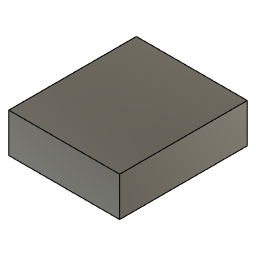
ConsoleFrame v17 (Autodesk Fusion 360 archive; units mm, degrees)
design "DAC Mock"
Autodesk Fusion 360 part; units mm, degrees
sketch "Sketch1" plane through (0, 0, 0) normal (0, 0, 1) x (1, 0, 0)
  line L0 (0, 0) -> (0, 65)
  line L1 (0, 65) -> (56.5, 65)
  line L2 (56.5, 65) -> (56.5, 0)
  line L3 (56.5, 0) -> (0, 0)
  dimension "d1" = 65
  dimension "d2" = 56.5
  constraint coincident L0.start L3.end
  constraint vertical L0
  constraint perpendicular L0 L1
  constraint perpendicular L1 L2
  constraint perpendicular L0 L3
  measures "d1" distance of L0.start L0.end
  measures "d2" distance of L0.end L1.end
extrude "Extrude1" add sketch "Sketch1" along normal blind 20

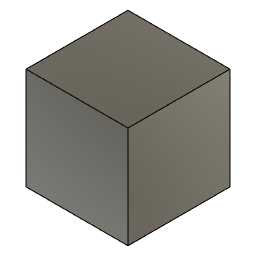
design "Relay Block"
Autodesk Fusion 360 part; units mm, degrees
sketch "Sketch1" plane through (0, 0, 0) normal (0, 0, 1) x (1, 0, 0)
  line L0 (0, 0) -> (0, 30)
  line L1 (0, 30) -> (30, 30)
  line L2 (30, 30) -> (30, 0)
  line L3 (30, 0) -> (0, 0)
  dimension "d1" = 30
  dimension "d2" = 30
  constraint coincident L0.start L3.end
  constraint vertical L0
  constraint perpendicular L0 L1
  constraint perpendicular L1 L2
  constraint perpendicular L0 L3
  measures "d1" distance of L0.start L0.end
  measures "d2" distance of L0.end L1.end
extrude "Extrude1" add sketch "Sketch1" along normal blind 30

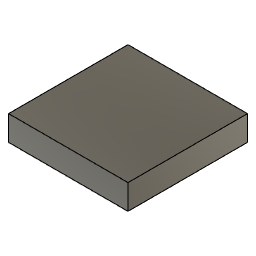
design "FanBlock"
Autodesk Fusion 360 part; units mm, degrees
sketch "Sketch1" plane through (0, 0, 0) normal (0, 0, 1) x (1, 0, 0)
  line L0 (0, 0) -> (0, 60) construction
  line L1 (0, 0) -> (60, 0) construction
  line L2 (0, 0) -> (-60, 0) construction
  line L3 (0, 60) -> (-60, 60)
  line L4 (-60, 60) -> (-60, -60)
  line L5 (-60, -60) -> (60, -60)
  line L6 (-60, 60) -> (60, 60)
  line L7 (60, 60) -> (60, -60)
  dimension "d1" = 60
  dimension "d2" = 60
  dimension "d3" = 60
  dimension "d4" = 120
  dimension "d5" = 120
  dimension "d6" = 120
  constraint coincident L0.start L1.start
  constraint vertical L0
  constraint perpendicular L0 L1
  constraint perpendicular L0 L2
  constraint perpendicular L0 L3
  constraint perpendicular L2 L4
  constraint horizontal L5
  constraint perpendicular L4 L6
  measures "d1" distance of L0.start L0.end
  measures "d2" distance of L0.start L1.end
  measures "d3" distance of L0.start L2.end
  measures "d4" distance of L3.end L4.end
  measures "d5" distance of L4.end L5.end
  measures "d6" distance of L3.end L6.end
extrude "Extrude1" add sketch "Sketch1" along normal blind 25

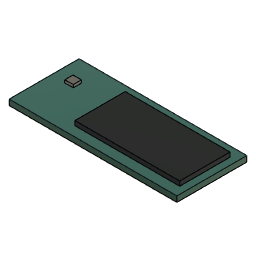
design "Adatrinket Power control"
Autodesk Fusion 360 part; units mm, degrees
sketch "Sketch1" plane through (0, 0, 0) normal (0, 0, 1) x (1, 0, 0)
  line L0 (0, 0) -> (0, 18)
  line L1 (0, 0) -> (37.5, 0)
  line L2 (0, 18) -> (37.5, 18)
  line L3 (37.5, 18) -> (37.5, 0)
  dimension "d1" = 18
  dimension "d2" = 37.5
  dimension "d3" = 37.5
  constraint coincident L0.start L1.start
  constraint vertical L0
  constraint perpendicular L0 L1
  constraint perpendicular L0 L2
  measures "d1" distance of L0.start L0.end
  measures "d2" distance of L0.start L1.end
  measures "d3" distance of L0.end L2.end
extrude "Extrude1" add sketch "Sketch1" along normal blind 1.6 makes body 1
move_body "Move1" bodies 1 to x (1, 0, 0) y (0, 1, 0) z (0, 0, 1) at (15, 0, 14)
sketch "Sketch2" plane through (0, 0, 0) normal (0, 0, 1) x (1, 0, 0)
  line L0 (0, 0) -> (60, 0)
  line L1 (60, 0) -> (60, 25)
  line L2 (60, 25) -> (0, 25)
  line L3 (0, 25) -> (0, 0)
  constraint coincident L0.start L3.end
  constraint horizontal L0
  constraint perpendicular L0 L1
  constraint perpendicular L1 L2
  constraint perpendicular L0 L3
extrude "Extrude2" add sketch "Sketch2" along normal blind 2 separate body makes body 2
move_body "Move2" bodies 1 to x (1, 0, 0) y (0, 1, 0) z (0, 0, 1) at (5, 0, -10)
move_body "Move3" bodies 1 to x (1, 0, 0) y (0, 1, 0) z (0, 0, 1) at (0, 3.5, 0)
sketch "Sketch3" plane through (0, 0, 2) normal (0, 0, 1) x (-1, 0, 0)
  line L0 (0, -25) -> (0, 0)
  line L1 (0, 0) -> (-60, 0)
  line L2 (-60, 0) -> (-60, -25)
  line L3 (-60, -25) -> (0, -25)
  line L4 (-4.9535, -17.884) -> (-4.9535, -14.884)
  line L5 (-4.9535, -17.884) -> (-7.9535, -17.884)
  line L6 (-7.9535, -17.884) -> (-7.9535, -15)
  line L7 (-7.9535, -15) -> (-4.9535, -14.884)
  dimension "d8" = 3
  dimension "d9" = 3
  constraint parallel L0 L4
  constraint perpendicular L4 L5
  constraint perpendicular L5 L6
  measures "d8" distance of L4.start L4.end
  measures "d9" distance of L4.start L5.end
extrude "Extrude3" add sketch "Sketch3" along normal blind 1 separate body contours L4 L5 L6 L7 makes body 3
sketch "Sketch4" plane through (0, 0, 2) normal (0, 0, 1) x (-1, 0, 0)
  line L0 (0, -25) -> (0, 0)
  line L1 (0, 0) -> (-60, 0)
  line L2 (-60, 0) -> (-60, -25)
  line L3 (-60, -25) -> (0, -25)
move_body "Move4" bodies 1 to x (1, 0, 0) y (0, 1, 0) z (0, 0, 1) at (0, 0, -2)

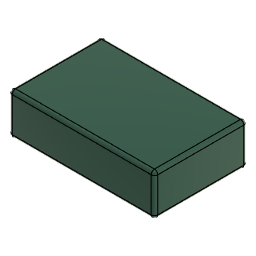
design "Rpi Standin"
Autodesk Fusion 360 part; units mm, degrees
sketch "Sketch1" plane through (0, 0, 0) normal (0, 0, 1) x (1, 0, 0)
  line L0 (0, 0) -> (0, 56)
  line L1 (0, 56) -> (88, 56)
  line L2 (0, 0) -> (88, 0)
  line L3 (88, 56) -> (88, 0)
  dimension "d1" = 56
  dimension "d2" = 88
  dimension "d3" = 88
  constraint coincident L0.start L2.start
  constraint vertical L0
  constraint perpendicular L0 L1
  constraint parallel L1 L2
  measures "d1" distance of L0.start L0.end
  measures "d2" distance of L0.end L1.end
  measures "d3" distance of L0.start L2.end
extrude "Extrude1" add sketch "Sketch1" along normal blind 25
fillet "Fillet1" radius 2 5 faces at (29.3333, 37.3333, 25) (29.3333, 56, 16.6667) (88, 37.3333, 8.3333) (29.3333, 0, 16.6667) (0, 18.6667, 8.3333)
